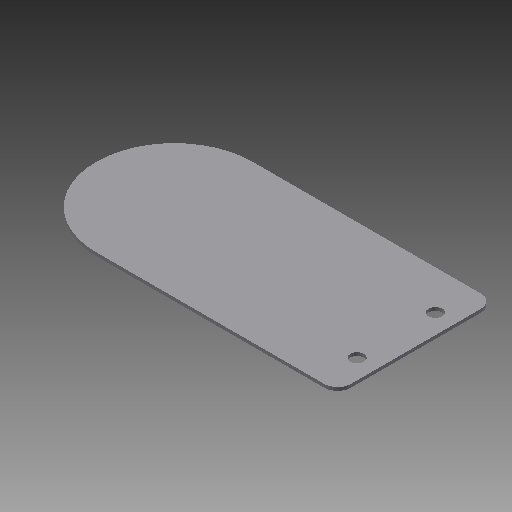
# Autodesk Inventor part: Türblech3
Saved by Autodesk Inventor 2018 (Build 220112000, 112)
## iProperties
Created: 2013-02-19
Part Number: Türblech3
Material: Generic
Document SubType Name: Modeling
Designer: Neef
Density: 1 g/cm^3
Appearance: Default
Author: Neef
Autodesk Inventor part; units mm, degrees
ref_plane "YZ Plane" through (0, 0, 0) normal (1, 0, 0) x (0, 1, 0)
ref_plane "XZ Plane" through (0, 0, 0) normal (0, 1, 0) x (-1, 0, 0)
ref_plane "XY Plane" through (0, 0, 0) normal (0, 0, 1) x (1, 0, 0)
sketch "Skizze1" plane through (0, 0, 0) normal (0, 0, 1) x (1, 0, 0)
  line L0 (0, 2.8971) -> (0, -17.3823) projected
  line L1 (-24.8652, 0) -> (47.7941, 0) projected
  line L2 (37, 0) -> (37, -10)
  line L3 (35, -12) -> (0, -12)
  arc A0 (-12, 0) -> (0, -12) centre (0, 0) ccw
  arc A1 (35, -12) -> (37, -10) centre (35, -10) ccw
  line L4 (-12, 0) -> (37, 0)
  point P0 (37, -12)
  dimension "d1" = 37
  dimension "d2" = 2
  dimension "d3" = 12
  constraints: 6 end point, 5 point on line, 4 point on circle, 3 tangent, 2 centre point, 2 perpendicular, 1 coincident, 1 collinear
  measures "d1" distance of point (37, -12) L3.end
  measures "d2" radius of A1
  measures "d3" radius of A0
extrude "Extrusion1" add sketch "Skizze1" along normal blind 0.5
mirror "Spiegeln1" about plane through (0, 0, 0) normal (0, 1, 0)
sketch "Skizze2" plane through (0, 0, 0.5) normal (0, 0, 1) x (1, 0, 0)
  line L0 (35, -12) -> (0, -12) projected
  line L1 (37, 10) -> (37, -10) projected
  point P0 (34, -6)
  dimension "d6" = 3
  dimension "d7" = 6
  measures "d6" distance from line of L1 point (34, -6)
  measures "d7" distance from line of L0 point (34, -6)
hole "Bohrung1" at (34, -6, 0.5) direction (0, 0, -1) diameter 2.1 end through all
mirror "Spiegeln2" about plane through (0, 0, 0) normal (0, 1, 0) of "Bohrung1"
